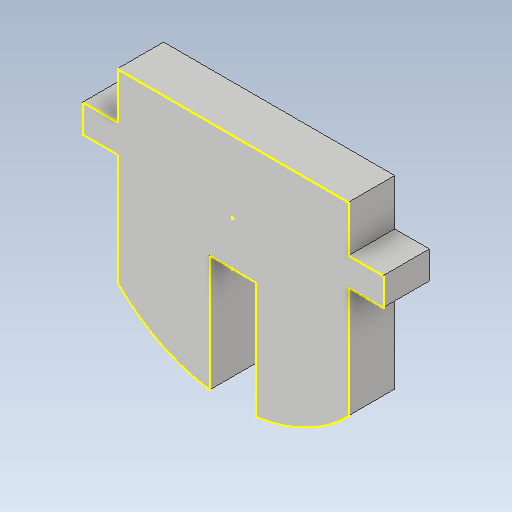
# Autodesk Inventor part: BottomPegCor
Saved by Autodesk Inventor 2020.1 (Build 241239000, 239)
## iProperties
Created: 2019-10-24
Part Number: BottomPegCor
Material: Generic
Document SubType Name: Modeling
Designer: j8qin
Density: 1 g/cm^3
Appearance: Default
Author: j8qin
Autodesk Inventor part; units mm, degrees
ref_plane "YZ Plane" through (0, 0, 0) normal (1, 0, 0) x (0, 1, 0)
ref_plane "XZ Plane" through (0, 0, 0) normal (0, 1, 0) x (-1, 0, 0)
ref_plane "XY Plane" through (0, 0, 0) normal (0, 0, 1) x (1, 0, 0)
sketch "Sketch1" plane through (0, 0, 0) normal (0, 0, 1) x (1, 0, 0)
  line L0 (-12.7, 7.62) -> (12.7, 7.62) construction
  line L1 (-12.7, -7.62) -> (12.7, 7.62) construction
  line L2 (-12.7, 7.62) -> (12.7, -7.62) construction
  line L3 (-6.35, -11.7818) -> (-6.35, 0) construction
  line L4 (-2.54, 0) -> (2.54, 0)
  line L5 (6.35, 0) -> (6.35, -11.7818) construction
  line L6 (-6.35, -12.954) -> (6.35, 0) construction
  line L7 (-6.35, 0) -> (6.35, -12.954) construction
  line L8 (-25.5271, -12.954) -> (-6.35, -12.954) construction
  line L9 (0, -12.954) -> (34.2013, -12.954) construction
  line L10 (-6.35, -7.62) -> (-12.7, -7.62) construction
  line L11 (12.7, -7.62) -> (6.35, -7.62) construction
  line L12 (-12.7, 7.62) -> (-12.7, 12.7)
  line L13 (-12.7, 12.7) -> (12.7, 12.7) construction
  line L14 (12.7, 12.7) -> (12.7, 7.62)
  arc A0 (-12.7, -7.62) -> (-6.35, -11.7818) centre (0, 4.832) ccw construction
  arc A1 (6.35, -11.7818) -> (12.7, -7.62) centre (0, 4.832) ccw
  line L15 (-12.7, 2.667) -> (-16.51, 2.667) construction
  line L16 (-16.51, 4.953) -> (-12.7, 4.953) construction
  line L17 (-8.89, 4.953) -> (-8.89, 2.667) construction
  line L18 (-8.89, 2.667) -> (-16.51, 4.953) construction
  line L19 (-16.51, 2.667) -> (-8.89, 4.953) construction
  line L20 (12.7, 2.667) -> (16.51, 2.667) construction
  line L21 (16.51, 4.953) -> (12.7, 4.953) construction
  line L22 (8.89, 4.953) -> (8.89, 2.667) construction
  line L23 (8.89, 2.667) -> (16.51, 4.953) construction
  line L24 (16.51, 2.667) -> (8.89, 4.953) construction
  line L25 (-12.7, -7.62) -> (-12.7, 2.286)
  line L26 (12.7, 2.286) -> (12.7, -7.62)
  line L27 (-12.7, 12.7) -> (12.7, 12.7)
  line L28 (-16.51, 4.953) -> (-16.51, 5.334)
  line L29 (6.35, 0) -> (5.715, 0) construction
  line L30 (-6.35, 0) -> (-5.715, 0) construction
  line L31 (-5.715, 0) -> (-5.715, -0.6477) construction
  line L32 (5.715, 0) -> (5.715, -0.6477) construction
  arc A2 (-6.35, -11.7818) -> (-5.715, -12.0108) centre (0, 4.832) ccw
  arc A3 (5.715, -12.0108) -> (6.35, -11.7818) centre (0, 4.832) ccw
  line L33 (-12.7, -7.62) -> (12.7, -7.62) construction
  line L34 (-5.715, 0) -> (-3.175, 0) construction
  line L35 (5.715, 0) -> (3.175, 0) construction
  arc A4 (-6.35, -11.7818) -> (-5.4965, -12.0834) centre (0, 4.832) ccw
  arc A5 (3.175, -12.6683) -> (12.7, -7.62) centre (0, 4.832) ccw
  line L36 (-12.7, 7.62) -> (-16.51, 7.62)
  line L37 (-16.51, 7.62) -> (-16.51, 4.572)
  line L38 (-16.51, 4.572) -> (-12.7, 4.572)
  line L39 (-12.7, 4.572) -> (-12.7, 1.9405)
  line L40 (12.7, 7.62) -> (16.51, 7.62)
  line L41 (16.51, 7.62) -> (16.51, 4.572)
  line L42 (16.51, 4.572) -> (12.7, 4.572)
  line L43 (12.7, 4.572) -> (12.7, 2.286)
  line L44 (-3.175, 0) -> (-2.54, 0) construction
  line L45 (-2.54, 0) -> (-2.54, -12.7717)
  line L46 (3.175, 0) -> (2.54, 0) construction
  line L47 (2.54, 0) -> (2.54, -12.7717)
  arc A6 (-12.7, -7.62) -> (-2.54, -12.7717) centre (0, 4.832) ccw
  arc A7 (2.54, -12.7717) -> (12.7, -7.62) centre (0, 4.832) ccw
  point P0 (0, 0)
  point P1 (0, -6.477)
  point P2 (-12.7, 3.81)
  point P3 (12.7, 3.81)
  dimension "d0" = 15.24
  dimension "d1" = 25.4
  dimension "d3" = 12.7
  dimension "d4" = 5.08
  dimension "d5" = 1.1722
  dimension "d7" = 7.62
  dimension "d8" = 2.286
  dimension "d9" = 7.62
  dimension "d17" = 0.635
  dimension "d18" = 0.635
  dimension "d19" = 90
  dimension "d22" = 2.54
  dimension "d24" = 2.54
  dimension "d30" = 3.81
  dimension "d31" = 3.048
  dimension "d33" = 3.81
  dimension "d36" = 0.635
  dimension "d37" = 0.635
  constraints: 96 end point, 16 point on circle, 11 perpendicular, 8 centre point, 8 midpoint, 6 horizontal, 6 parallel, 6 point on line, 4 vertical, 2 collinear, 2 tangent
  measures "d0" distance of L1.start L0.start
  measures "d1" distance of L0.start L0.end
  measures "d3" distance of L3.end L5.start
  measures "d4" distance of L0.start L12.end
  measures "d5" distance of L3.start L6.start
  measures "d7" distance of L17.end L15.end
  measures "d8" distance of L15.end L16.start
  measures "d9" distance of L22.end L20.end
  measures "d17" distance of L29.end L5.start
  measures "d18" distance of L30.end L3.end
  measures "d19" angle of L30 L31
  measures "d22" distance of L34.end L30.end
  measures "d24" distance of L35.end L29.end
  measures "d30" distance of L0.start L36.end
  measures "d31" distance of L36.end L37.end
  measures "d33" distance of L0.end L40.end
  measures "d36" distance of L4.start L34.end
  measures "d37" distance of L4.end L35.end
extrude "Extrusion6" add sketch "Sketch1" along normal mid plane 5.08
sketch "Sketch2" plane through (0, 0, 2.54) normal (0, 0, 1) x (1, 0, 0)
  line L0 (-12.7, 4.572) -> (-12.7, -7.62) projected
  arc A0 (-12.7, -7.62) -> (-2.54, -12.7717) centre (0, 4.832) ccw projected
  line L1 (-2.54, -12.7717) -> (-2.54, 0) projected
  line L2 (-2.54, 0) -> (2.54, 0) projected
  line L3 (2.54, 0) -> (2.54, -12.7717) projected
  arc A1 (2.54, -12.7717) -> (12.7, -7.62) centre (0, 4.832) ccw projected
  line L4 (12.7, -7.62) -> (12.7, 4.572) projected
  line L5 (12.7, 4.572) -> (16.51, 4.572) projected
  line L6 (16.51, 4.572) -> (16.51, 7.62) projected
  line L7 (16.51, 7.62) -> (12.7, 7.62) projected
  line L8 (12.7, 7.62) -> (12.7, 12.7) projected
  line L9 (12.7, 12.7) -> (-12.7, 12.7) projected
  line L10 (-12.7, 12.7) -> (-12.7, 7.62) projected
  line L11 (-12.7, 7.62) -> (-16.51, 7.62) projected
  line L12 (-16.51, 7.62) -> (-16.51, 4.572) projected
  line L13 (-16.51, 4.572) -> (-12.7, 4.572) projected
  point P0 (0, 0)
body "Solid6"
